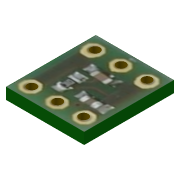
# Autodesk Inventor part: chip_gross
Saved by Autodesk Inventor 2017 (Build 210142000, 142)
## iProperties
Part Number: chip_gross
Material: Generisch
Document SubType Name: Modeling
Designer: Philomena-Theresa
Density: 1 g/cm^3
Appearance: Vorgabe
Author: Philomena-Theresa
Autodesk Inventor part; units mm, degrees
ref_plane "YZ Plane" through (0, 0, 0) normal (1, 0, 0) x (0, 1, 0)
ref_plane "XZ Plane" through (0, 0, 0) normal (0, 1, 0) x (-1, 0, 0)
ref_plane "XY Plane" through (0, 0, 0) normal (0, 0, 1) x (1, 0, 0)
sketch "Skizze1" plane through (0, 0, 0) normal (0, 0, 1) x (1, 0, 0)
  line L0 (-3.85, 4.425) -> (3.85, 4.425)
  line L1 (3.85, 4.425) -> (3.85, -4.425)
  line L2 (3.85, -4.425) -> (-3.85, -4.425)
  line L3 (-3.85, -4.425) -> (-3.85, 4.425)
  line L4 (-3.85, 4.425) -> (3.85, -4.425) construction
  point P0 (0, 0)
  point P1 (0, 0)
  dimension "d0" = 7.7
  dimension "d1" = 8.85
  constraints: 10 end point, 2 parallel, 1 coincident, 1 horizontal, 1 midpoint, 1 perpendicular
  measures "d0" distance of L1.end L2.end
  measures "d1" distance of L0.end L1.end
extrude "Extrusion2" add sketch "Skizze1" along normal blind 1.11
sketch "Skizze2" plane through (0, 0, 1.11) normal (0, 0, 1) x (1, 0, 0)
  line L0 (3.85, 4.425) -> (-3.85, 4.425) construction
  line L1 (-3.85, 4.425) -> (-3.85, 3.125) construction
  line L2 (-3.85, 4.425) -> (-3.85, -4.425) construction
  line L3 (-3.85, 3.125) -> (3.85, 3.125) construction
  line L4 (3.85, -4.425) -> (3.85, 4.425) construction
  line L5 (-3.85, 3.125) -> (-3.05, 3.125) construction
  line L6 (3.85, 3.125) -> (3.05, 3.125) construction
  line L7 (-3.05, 3.125) -> (-2.6, 3.125) construction
  circle A0 centre (-2.6, 3.125) radius 0.45
  circle A1 centre (-0.05, 3.125) radius 0.45
  circle A2 centre (2.5, 3.125) radius 0.45
  circle A3 centre (5.05, 3.125) radius 0.45
  circle A4 centre (7.6, 3.125) radius 0.45
  circle A5 centre (10.15, 3.125) radius 0.45
  line L8 (-3.85, -4.425) -> (-3.85, -3.125) construction
  line L9 (-3.85, -3.125) -> (3.85, -3.125) construction
  line L10 (-3.85, -3.125) -> (-2.6, -3.125) construction
  circle A6 centre (-2.6, -3.125) radius 0.45
  circle A7 centre (-0.05, -3.125) radius 0.45
  line L11 (-1.3, -3.125) -> (6.4, -3.125) construction
  circle A8 centre (2.5, -3.125) radius 0.45
  line L12 (1.25, -3.125) -> (8.95, -3.125) construction
  circle A9 centre (5.05, -3.125) radius 0.45
  line L13 (3.8, -3.125) -> (11.5, -3.125) construction
  circle A10 centre (7.6, -3.125) radius 0.45
  line L14 (6.35, -3.125) -> (14.05, -3.125) construction
  circle A11 centre (10.15, -3.125) radius 0.45
  line L15 (8.9, -3.125) -> (16.6, -3.125) construction
  line L16 (3.05, 3.125) -> (2.6, 3.125)
  point P0 (0, 0)
  dimension "d6" = 1.3
  dimension "d7" = 0.8
  dimension "d8" = 0.8
  dimension "d9" = 0.45
  dimension "d10" = 0.9
  dimension "d13" = 2.55
  dimension "d20" = 1.3
  dimension "d21" = 1.25
  dimension "d22" = 0.9
  dimension "d25" = 2.55
  dimension "d30" = 0.45
  constraints: 28 end point, 14 point on line, 12 centre point, 9 coincident, 2 horizontal, 2 perpendicular, 1 collinear, 39 other
  measures "d6" distance of L0.end L1.end
  measures "d7" distance of L1.end L5.end
  measures "d8" distance of L3.end L6.end
  measures "d9" distance of L7.start L7.end
  measures "d10" diameter of A0
  measures "d13" distance of A0.centre A1.centre
  measures "d20" distance of L2.end L8.end
  measures "d21" distance of L8.end L10.end
  measures "d22" diameter of A6
  measures "d25" distance of A6.centre A7.centre
  measures "d30" distance of L16.start L16.end
extrude "Extrusion3" cut sketch "Skizze2" against normal blind 1.11 contours A0 | A1 | A2 | A3 | A4 | A5 | A6 | A7 | A8 | A10 | A11
sketch "Skizze3" plane through (0, 0, 1.11) normal (0, 0, 1) x (1, 0, 0)
  line L0 (3.8509, -4.4242) -> (-3.85, -4.425) construction
  line L1 (-3.85, -4.425) -> (-3.8509, 4.4242) construction
  line L2 (-3.8509, 4.4242) -> (3.85, 4.425) construction
  line L3 (3.85, 4.425) -> (3.8509, -4.4242) construction
  point P0 (0, 0)
  point P1 (3.85, 4.425)
  point P2 (-3.85, -4.425)
  constraints: 2 coincident, 2 other
decal "Aufkleber1"
